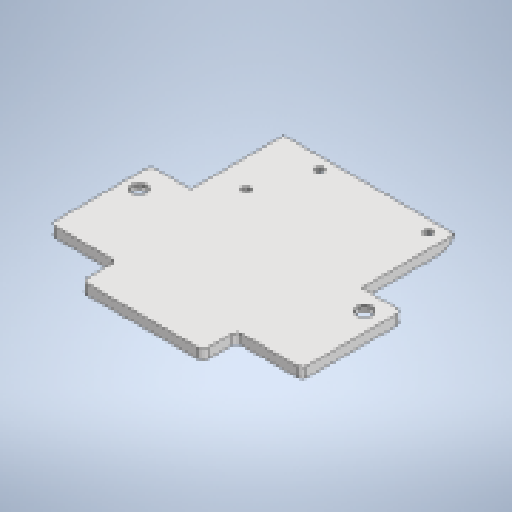
# Autodesk Inventor part: podstawa_v2
Saved by Autodesk Inventor 2023.5 (Build 275446000, 446)
## iProperties
Created: 2025-03-17
Part Number: podstawa_v2
Material: Ogólny
Document SubType Name: Modeling
Designer: kamil
Density: 1 g/cm^3
Appearance: Domyślna
Author: kamil
Autodesk Inventor part; units mm, degrees
ref_plane "YZ Plane" through (0, 0, 0) normal (1, 0, 0) x (0, 1, 0)
ref_plane "XZ Plane" through (0, 0, 0) normal (0, 1, 0) x (-1, 0, 0)
ref_plane "XY Plane" through (0, 0, 0) normal (0, 0, 1) x (1, 0, 0)
sketch "Szkic1" plane through (0, 0, 0) normal (0, 1, 0) x (-1, 0, 0)
  line L0 (0, 0) -> (-50, 0)
  line L1 (-50, 0) -> (-50, -50)
  line L2 (-50, -50) -> (0, -50)
  line L3 (0, -50) -> (0, 0)
  line L4 (0, -50) -> (-8, -50)
  line L5 (-8, -50) -> (-8, -30)
  line L6 (-8, -30) -> (0, -30)
  line L7 (0, -30) -> (0, -50)
  line L8 (-50, -50) -> (-42, -50)
  line L9 (-42, -50) -> (-42, -30)
  line L10 (-42, -30) -> (-50, -30)
  line L11 (-50, -30) -> (-50, -50)
  dimension "d0" = 50
  dimension "d1" = 50
  dimension "d2" = 8
  dimension "d3" = 20
  dimension "d4" = 8
  dimension "d5" = 20
  constraints: 24 end point, 6 parallel, 3 horizontal, 3 perpendicular, 1 coincident
  measures "d0" distance of L2.end L1.end
  measures "d1" distance of L1.end L0.end
  measures "d2" distance of L5.end L6.end
  measures "d3" distance of L4.end L5.end
  measures "d4" distance of L10.end L9.end
  measures "d5" distance of L9.end L8.end
extrude "Wyciągnięcie proste1" add sketch "Szkic1" along normal blind 2 contours L3 L6 L5 L2 L9 L10 L1 L0
sketch "Szkic4" plane through (0, 2, 0) normal (0, 1, 0) x (1, 0, 0)
  line L0 (42, 50) -> (8, 50) projected
  line L1 (12.0571, 48.5) -> (42.467, 48.5) projected
  line L2 (42, 30) -> (42, 50) projected
  line L3 (42, 50) -> (8, 50)
  line L4 (8, 50) -> (8, 48.5)
  line L5 (8, 48.5) -> (42, 48.5)
  line L6 (42, 48.5) -> (42, 50)
  circle A0 centre (39.467, 46.75) radius 0.85 projected
  circle A1 centre (15.0571, 46.75) radius 0.85 projected
  arc A2 (48.301, 27.6749) -> (46.5, 27.9321) centre (47.25, 26.75) ccw projected
  point P0 (0, 0)
  point P1 (42, 48.5)
  constraints: 8 end point, 2 parallel, 1 horizontal, 1 perpendicular
extrude "Wyciągnięcie proste3" cut sketch "Szkic4" against normal through all
sketch "Szkic6" plane through (0, 0, -30) normal (-1, 0, 0) x (0, 0, 1)
  line L0 (0, 0) -> (30, 0) projected
  line L1 (30, 0) -> (30, 2) projected
  line L2 (0, 2) -> (30, 2) projected
  line L3 (0, 0) -> (0, 2) projected
  line L4 (20.8419, 34.4275) -> (27.9622, -2) projected
  line L5 (27.9622, -2) -> (30, -2) projected
  line L6 (30, -2) -> (22.8048, 34.8111) projected
  line L7 (22.8048, 34.8111) -> (20.8419, 34.4275) projected
  point P0 (27.1803, 2)
  point P1 (27.5712, 0)
extrude "Wyciągnięcie proste5" cut sketch "Szkic6" against normal through all contours L4 L2 L6 L0 | L6 L2 L1 L0
sketch "Szkic7" plane through (0, 0, 0) normal (0, -1, 0) x (1, 0, 0)
  line L0 (50, -2.4288) -> (0, -2.4288) projected
  line L1 (0, -30) -> (0, -2.4288) projected
  line L2 (8, -30) -> (0, -30) projected
  line L3 (8, -48.5) -> (8, -30) projected
  line L4 (8, -48.5) -> (42, -48.5) projected
  line L5 (42, -30) -> (42, -48.5) projected
  line L6 (50, -30) -> (42, -30) projected
  line L7 (50, -2.4288) -> (50, -30) projected
  circle A0 centre (39.467, -46.75) radius 0.85 projected
  circle A1 centre (15.0571, -46.75) radius 0.85 projected
  line L8 (4, -10.1324) -> (0, -10.1324) projected
  line L9 (50, -10.1324) -> (45.5, -10.1324) projected
  line L10 (50, -10.1324) -> (42, -10.1324)
  line L11 (42, -10.1324) -> (42, -2.4288)
  line L12 (42, -2.4288) -> (50, -2.4288)
  line L13 (50, -2.4288) -> (50, -10.1324)
  line L14 (0, -2.4288) -> (8, -2.4288)
  line L15 (8, -2.4288) -> (8, -10.1324)
  line L16 (8, -10.1324) -> (0, -10.1324)
  line L17 (0, -10.1324) -> (0, -2.4288)
  point P0 (0, 0)
  dimension "d16" = 8
  dimension "d17" = 8
  constraints: 16 end point, 4 parallel, 2 horizontal, 2 perpendicular, 1 collinear, 1 point on line
  measures "d16" distance between parallel lines of L13 L11
  measures "d17" distance of L15.end L16.end
extrude "Wyciągnięcie proste6" cut sketch "Szkic7" against normal through all contours L7 L9 L10 L11 L0 | L15 L16 L8 L1 L0
fillet "Zaokrąglenie1" radius 1 4 edges at (0, 1, -30) (0, 1, -10.1324) (50, 1, -10.1324) (50, 1, -30)
sketch "Szkic9" plane through (0, 2, 0) normal (0, 1, 0) x (1, 0, 0)
  circle A0 centre (15.0571, 46.75) radius 0.85 projected
  circle A1 centre (39.467, 46.75) radius 0.85 projected
  point P0 (0, 0)
extrude "Wyciągnięcie proste8" add sketch "Szkic9" against normal up to surface (2 mm away)
sketch "Szkic10" plane through (0, 0, 0) normal (0, -1, 0) x (1, 0, 0)
  circle A0 centre (17.4483, -46.15) radius 0.6 projected
  circle A1 centre (39.0758, -46.15) radius 0.6 projected
  circle A2 centre (13.5571, -35.5) radius 0.6 projected
  circle A3 centre (46.2335, -26.3) radius 1.35 projected
  circle A4 centre (47.3, -13.0919) radius 1.35 projected
  circle A5 centre (3, -27) radius 1.4 projected
  circle A6 centre (3, -27) radius 1.55
  circle A7 centre (46.2335, -26.3) radius 1.55
  circle A8 centre (47.3, -13.0919) radius 1.55
  circle A9 centre (13.5571, -35.5) radius 0.85
  circle A10 centre (17.4483, -46.15) radius 0.85
  circle A11 centre (39.0758, -46.15) radius 0.85
  point P0 (0, 0)
  dimension "d25" = 3.1
  dimension "d26" = 1.7
  constraints: 6 centre point, 6 coincident, 4 equal radius
  measures "d25" diameter of A6
  measures "d26" diameter of A9
extrude "Wyciągnięcie proste9" cut sketch "Szkic10" against normal through all contours A0 | A1 | A2 | A3 | A7 | A9 | A10 | A11
sketch "Szkic11" plane through (0, 0, 0) normal (0, -1, 0) x (1, 0, 0)
  circle A0 centre (47.3, -13.0919) radius 1.55 projected
  circle A1 centre (46.2335, -26.3) radius 1.55 projected
  circle A2 centre (3, -27) radius 1.55 projected
  circle A3 centre (13.5571, -35.5) radius 0.85 projected
  circle A4 centre (17.4483, -46.15) radius 0.85 projected
  circle A5 centre (39.0758, -46.15) radius 0.85 projected
  point P0 (0, 0)
hole "Otwór1" at (46.2335, 0, -26.3) direction (0, 1, 0) diameter 5 depth 1.1
hole "Otwór2" at (13.5571, 0, -35.5) at (17.4483, 0, -46.15) at (39.0758, 0, -46.15) direction (0, 1, 0) diameter 3 depth 1
sketch "Szkic12" plane through (0, 0, 0) normal (0, -1, 0) x (1, 0, 0)
  line L0 (49, -10.1324) -> (42, -10.1324) projected
  line L1 (8, -10.1324) -> (1, -10.1324) projected
  line L2 (50, -11.1324) -> (50, -29) projected
  line L3 (0, -29) -> (0, -11.1324) projected
  line L4 (50, -2.4288) -> (37, -2.4288)
  line L5 (37, -2.4288) -> (37, -10.1324)
  line L6 (37, -10.1324) -> (50, -10.1324)
  line L7 (50, -10.1324) -> (50, -2.4288)
  line L8 (0, -2.4288) -> (13, -2.4288)
  line L9 (13, -2.4288) -> (13, -10.1324)
  line L10 (13, -10.1324) -> (0, -10.1324)
  line L11 (0, -10.1324) -> (0, -2.4288)
  line L12 (42, -2.4288) -> (8, -2.4288) projected
  point P0 (0, 0)
  dimension "d43" = 13
  dimension "d44" = 13
  constraints: 16 end point, 6 collinear, 4 parallel, 2 horizontal, 2 perpendicular
  measures "d43" distance between parallel lines of L7 L5
  measures "d44" distance of L8.start L8.end
extrude "Wyciągnięcie proste10" cut sketch "Szkic12" against normal through all
fillet "Zaokrąglenie2" radius 1 2 edges at (13, 1, -10.1324) (37, 1, -10.1324)
sketch "Szkic13" plane through (0, 2, 0) normal (0, 1, 0) x (1, 0, 0)
  line L0 (10.7953, -1.4378) -> (38.6557, -1.4378)
  line L1 (38.6557, -1.4378) -> (38.6557, 3.4288)
  line L2 (38.6557, 3.4288) -> (10.7953, 3.4288)
  line L3 (10.7953, 3.4288) -> (10.7953, -1.4378)
  line L4 (37, 2.4288) -> (13, 2.4288) projected
  point P0 (0, 0)
  dimension "d48" = 1
  constraints: 8 end point, 2 parallel, 1 horizontal, 1 perpendicular
  measures "d48" distance between parallel lines of L2 L4
extrude "Wyciągnięcie proste11" cut sketch "Szkic13" against normal through all
fillet "Zaokrąglenie3" radius 1 2 edges at (13, 1, -3.4288) (37, 1, -3.4288)
fillet "Zaokrąglenie4" radius 4 1 edges at (25, 0, -48.5)
chamfer "Faza1" distance 0.5 angle 45 4 edges at (16.5983, 1, -46.15) (38.2258, 1, -46.15) (44.6835, 1.1, -26.3) (12.7071, 1, -35.5)
sketch "Szkic14" plane through (0, 0, 0) normal (0, -1, 0) x (1, 0, 0)
  circle A0 centre (2.8, -24.8689) radius 1.4 projected
  point P0 (0, 0)
hole "Otwór3" at (2.8, 0, -24.8689) direction (0, 1, 0) diameter 3 depth 2 counterbore diameter 5 counterbore depth 1
chamfer "Faza2" distance 0.5 angle 45 1 edges at (2.8, 1, -23.3689)
